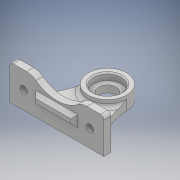
# Autodesk Inventor part: holder-bearing-z-axis
Saved by Autodesk Inventor 2018 (Build 220112000, 112)
## iProperties
Created: 2017-11-04
Part Number: holder-bearing-z-axis
Material: Generic
Document SubType Name: Modeling
Designer: Jurjen
Density: 1 g/cm^3
Appearance: Default
Author: Jurjen
Autodesk Inventor part; units mm, degrees
ref_plane "YZ Plane" through (0, 0, 0) normal (1, 0, 0) x (0, 1, 0)
ref_plane "XZ Plane" through (0, 0, 0) normal (0, 1, 0) x (-1, 0, 0)
ref_plane "XY Plane" through (0, 0, 0) normal (0, 0, 1) x (1, 0, 0)
sketch "Sketch1" plane through (0, 0, 0) normal (0, 0, 1) x (1, 0, 0)
  circle A0 centre (0, 14.8408) radius 5
  arc A1 (11, 14.8408) -> (-11, 14.8408) centre (0, 14.8408) ccw
  arc A2 (-27, -10.1592) -> (-11, 14.8408) centre (-38.5312, 14.8408) ccw
  line L0 (-27, -10.1592) -> (-27, -14.1592)
  line L1 (-27, -14.1592) -> (0, -14.1592)
  line L2 (0, -14.1592) -> (0, 0) construction
  arc A3 (11, 14.8408) -> (27, -10.1592) centre (38.5312, 14.8408) ccw
  line L3 (27, -10.1592) -> (27, -14.1592)
  line L4 (27, -14.1592) -> (0, -14.1592)
  arc A4 (-11, 14.8408) -> (11, 14.8408) centre (0, 14.8408) ccw construction
  point P0 (-15.3425, 0)
  dimension "d0" = 10
  dimension "d1" = 22
  dimension "d2" = 4
  dimension "d3" = 27
  dimension "d4" = 25
  constraints: 10 end point, 9 point on circle, 5 centre point, 4 symmetric about line, 2 horizontal alignment, 2 vertical, 2 vertical alignment, 1 coincident, 1 perpendicular, 1 tangent, 1 other
  measures "d0" diameter of A0
  measures "d1" diameter of A1
  measures "d2" distance of L0.start L0.end
  measures "d3" distance of L1.end L0.end
  measures "d4" vertical distance of A0.centre L0.start
extrude "Extrusion1" add sketch "Sketch1" along normal mid plane 4
sketch "Sketch2" plane through (0, 0, 2) normal (0, 0, 1) x (1, 0, 0)
  circle A0 centre (0, 14.8408) radius 5 projected
  arc A1 (11, 14.8408) -> (-11, 14.8408) centre (0, 14.8408) ccw projected
  circle A2 centre (0, 14.8408) radius 11
  circle A3 centre (0, 14.8408) radius 8
  point P0 (0, 0)
  dimension "d7" = 16
  constraints: 2 coincident, 1 centre point, 1 horizontal alignment, 2 other
  measures "d7" diameter of A3
extrude "Extrusion2" add sketch "Sketch2" along normal blind 4 contours A2 A1
sketch "Sketch3" plane through (0, 0, 2) normal (0, 0, 1) x (1, 0, 0)
  line L0 (-27, -14.1592) -> (27, -14.1592) projected
  line L1 (-27, -10.1592) -> (-27, -14.1592) projected
  line L2 (27, -14.1592) -> (-27, -14.1592)
  line L3 (-27, -14.1592) -> (-27, -10.1592)
  line L4 (-27, -10.1592) -> (27, -10.1592)
  line L5 (27, -10.1592) -> (27, -14.1592)
  point P0 (0, 0)
  constraints: 8 end point, 2 parallel, 1 horizontal, 1 perpendicular
extrude "Extrusion3" add sketch "Sketch3" along normal blind 16
sketch "Sketch4" plane through (-27, -10.1592, 2) normal (0, 1, 0) x (1, 0, 0)
  circle A0 centre (46, -6) radius 2.1
  circle A1 centre (8, -6) radius 2.1
  line L0 (54, -16) -> (0, -16) projected
  line L1 (54, 0) -> (54, -16) projected
  line L2 (0, 0) -> (0, -16) projected
  point P0 (27, 2)
  dimension "d12" = 4.2
  dimension "d13" = 10
  dimension "d14" = 8
  dimension "d15" = 8
  constraints: 2 centre point, 1 equal radius, 1 horizontal alignment
  measures "d12" diameter of A0
  measures "d13" distance from line of L0 A0.centre
  measures "d14" distance from line of L1 A0.centre
  measures "d15" distance from line of L2 A1.centre
extrude "Extrusion4" cut sketch "Sketch4" against normal up to next
fillet "Fillet1" radius 2 4 edges at (27, -12.1592, 18) (-27, -12.1592, 18) (0, -10.1592, 2) (0, 3.8408, 2)
chamfer "Chamfer1" distance 0.7 angle 45 1 edges at (-8, 14.8408, 6)
sketch "Sketch5" plane through (-27, -14.1592, -2) normal (0, -1, 0) x (1, 0, 0)
  line L0 (17, 11.25) -> (37, 11.25)
  line L1 (37, 11.25) -> (37, 8.75)
  line L2 (37, 8.75) -> (17, 8.75)
  line L3 (17, 8.75) -> (17, 11.25)
  circle A0 centre (46, 10) radius 2.1 projected
  circle A1 centre (8, 10) radius 2.1 projected
  point P0 (27, 2)
  point P1 (17, 10)
  point P2 (27, 11.25)
  dimension "d22" = 2.5
  dimension "d23" = 20
  constraints: 8 end point, 2 midpoint, 2 parallel, 1 horizontal, 1 horizontal alignment, 1 perpendicular, 1 vertical alignment
  measures "d22" distance of L0.end L1.end
  measures "d23" distance between parallel lines of L1 L3
extrude "Extrusion5" add sketch "Sketch5" along normal blind 2 contours L0 L1 L2 L3
chamfer "Chamfer2" distance 2 angle 45 4 edges at (0, -14.1592, 6.75) (0, -14.1592, 9.25) (-10, -14.1592, 8) (10, -14.1592, 8)
sketch "Sketch6" plane through (-27, -10.1592, 4) normal (0, 1, 0) x (1, 0, 0)
  line L0 (52, -14) -> (2, -14) projected
  arc A0 (41, -14) -> (13, -14) centre (27, -28.2829) ccw
  point P0 (27, 4)
  point P1 (27, -8.2829)
  point P2 (27, -14)
  dimension "d29" = 20
  dimension "d30" = 14
  constraints: 3 point on circle, 2 point on line, 1 centre point, 1 midpoint, 1 vertical alignment
  measures "d29" radius of A0
  measures "d30" distance of A0.end point (27, -14)
extrude "Extrusion6" cut sketch "Sketch6" against normal up to next
fillet "Fillet2" radius 9 2 edges at (14, -12.1592, 18) (-14, -12.1592, 18)
equation "\"d15\" = d14"
body "Solid1"
